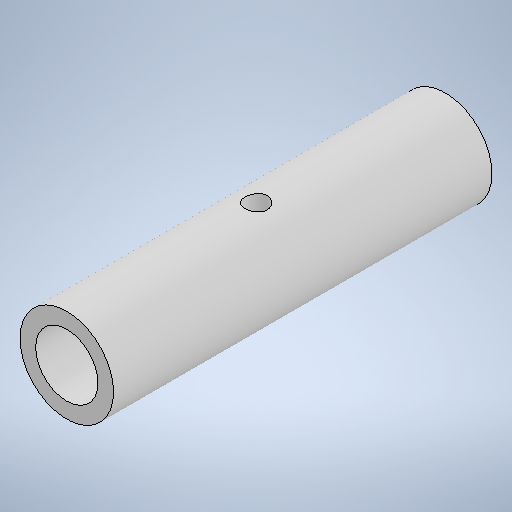
# Autodesk Inventor part: 212.1
Saved by Autodesk Inventor 2025 (Build 290162010, 162A)
## iProperties
Created: 2024-06-09
Part Number: 212.1
Material: Generic
Document SubType Name: Modeling
Designer: Fabri
Density: 1 g/cm^3
Appearance: Default
Author: Fabri
Autodesk Inventor part; units mm, degrees
ref_plane "YZ Plane" through (0, 0, 0) normal (1, 0, 0) x (0, 1, 0)
ref_plane "XZ Plane" through (0, 0, 0) normal (0, 1, 0) x (-1, 0, 0)
sketch "Sketch1" plane through (0, 0, 0) normal (0, 1, 0) x (-1, 0, 0)
  circle A0 centre (0, 0) radius 10.5
  circle A1 centre (0, 0) radius 7
  dimension "d0" = 21
  dimension "d1" = 14
  constraints: 2 centre point, 2 coincident
  measures "d0" diameter of A0
  measures "d1" diameter of A1
extrude "Extrusion1" add sketch "Sketch1" along normal blind 85
ref_plane "Work Plane1" through (0, 0, -10.75) normal (0, 0, -1) x (-1, 0, 0)
sketch "Sketch2" plane through (0, 0, -10.75) normal (0, 0, -1) x (-1, 0, 0)
  line L0 (10.5, 0) -> (-10.5, 0) projected
  point P0 (0, 0)
  point P1 (0, 42.5)
  dimension "d5" = 42.5
  constraints: 1 vertical alignment
  measures "d5" distance from line of point (0, 42.5) L0
hole "Hole1" at (0, 42.5, -10.75) direction (0, 0, 1) diameter 5 end through all
body "Solid1"
